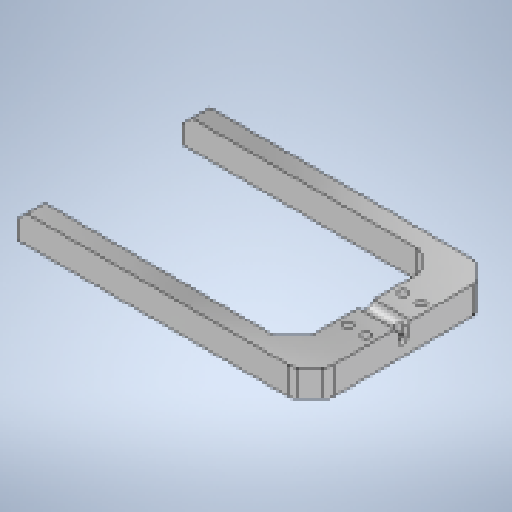
# Autodesk Inventor part: Rack
Saved by Autodesk Inventor 2023.2 (Build 272271000, 271)
## iProperties
Created: 2024-01-11
Part Number: Rack
Material: Aluminum 6061
Document SubType Name: Modeling
Designer: Nathan Cai
Mass: 47.5028 g
Surface Area: 86.9372 cm^2
Volume: 17.5936 cm^3
Density: 2.7 g/cm^3
Appearance: Aluminum - Flat
Author: Nathan Cai
Autodesk Inventor part; units mm, degrees
ref_plane "YZ Plane" through (0, 0, 0) normal (1, 0, 0) x (0, 1, 0)
ref_plane "XZ Plane" through (0, 0, 0) normal (0, 1, 0) x (-1, 0, 0)
ref_plane "XY Plane" through (0, 0, 0) normal (0, 0, 1) x (1, 0, 0)
sketch "Sketch1" plane through (0, 0, 0) normal (0, 1, 0) x (-1, 0, 0)
  line L0 (44.45, 23.8125) -> (-44.45, 23.8125)
  line L1 (-44.45, 23.8125) -> (-44.45, -23.8125)
  line L2 (-44.45, -23.8125) -> (44.45, -23.8125)
  line L3 (44.45, -23.8125) -> (44.45, 23.8125)
  line L4 (44.45, 23.8125) -> (-44.45, -23.8125) construction
  line L5 (-44.45, 23.8125) -> (44.45, -23.8125) construction
  line L6 (0, 0) -> (-44.45, 0) construction
  line L7 (44.45, 30.1625) -> (-57.15, 30.1625)
  line L8 (-57.15, 30.1625) -> (-57.15, -30.1625)
  line L9 (-57.15, -30.1625) -> (44.45, -30.1625)
  line L10 (44.45, -30.1625) -> (44.45, 30.1625)
  line L11 (44.45, 30.1625) -> (-57.15, -30.1625) construction
  line L12 (-57.15, 30.1625) -> (44.45, -30.1625) construction
  point P0 (-6.35, 0)
  point P1 (44.45, 23.8125)
  dimension "d0" = 88.9
  dimension "d1" = 47.625
  dimension "d2" = 6.35
  dimension "d3" = 12.7
  constraints: 26 end point, 5 midpoint, 4 parallel, 2 horizontal, 2 perpendicular, 2 point on line
  measures "d0" distance of L2.end L1.end
  measures "d1" distance of L1.end L0.end
  measures "d2" distance between parallel lines of L2 L9
  measures "d3" distance between parallel lines of L1 L8
extrude "Extrusion1" add sketch "Sketch1" along normal blind 9.525 contours L0 L1 L2 L10 L9 L8 L7
chamfer "Chamfer1" distance 6.35 angle 45 4 edges at (44.45, 4.7625, 23.8125) (57.15, 4.7625, 30.1625) (44.45, 4.7625, -23.8125) (57.15, 4.7625, -30.1625)
fillet "Fillet1" radius 3.175 8 edges at (38.1, 4.7625, 23.8125) (44.45, 4.7625, 17.4625) (44.45, 4.7625, -17.4625) (38.1, 4.7625, -23.8125) (50.8, 4.7625, -30.1625) (57.15, 4.7625, -23.8125) (57.15, 4.7625, 23.8125) (50.8, 4.7625, 30.1625)
sketch "Sketch2" plane through (57.15, 0, 22.4974) normal (1, 0, 0) x (0, 0, -1)
  line L0 (38.6447, 9.525) -> (6.35, 9.525) projected
  line L1 (22.4974, 9.525) -> (22.4974, 0) construction
  line L2 (38.6447, 0) -> (6.35, 0) projected
  circle A0 centre (22.4974, 4.7625) radius 3.175 construction
  circle A1 centre (22.4974, 11.1125) radius 3.175
  line L3 (22.4974, 17.1125) -> (22.4974, 5.1125) construction
  line L4 (20.9974, 17.1125) -> (20.9974, 5.1125)
  line L5 (23.9974, 5.1125) -> (23.9974, 17.1125)
  arc A2 (23.9974, 17.1125) -> (20.9974, 17.1125) centre (22.4974, 17.1125) ccw
  arc A3 (20.9974, 5.1125) -> (23.9974, 5.1125) centre (22.4974, 5.1125) ccw
  point P0 (19.7477, 9.525)
  point P1 (25.247, 9.525)
  point P2 (23.9974, 8.3142)
  point P3 (20.9974, 8.3142)
  dimension "d10" = 6.35
  dimension "d20" = 6.35
  dimension "d21" = 6.35
  dimension "d22" = 3
  dimension "d23" = 12
  constraints: 10 end point, 4 centre point, 4 point on circle, 4 tangent, 3 midpoint, 2 point on line, 1 parallel, 1 perpendicular
  measures "d10" diameter of A0
  measures "d20" diameter of A1
  measures "d21" distance of A0.centre A1.centre
  measures "d22" diameter of A3
  measures "d23" distance of L3.end L3.start
sketch "Sketch4" plane through (0, 9.525, 0) normal (0, 1, 0) x (1, 0, 0)
  line L0 (44.45, 16.1474) -> (44.45, -16.1474) projected
  line L1 (44.45, 0) -> (57.15, 0) construction
  line L2 (57.15, -22.4974) -> (57.15, 22.4974) projected
  line L3 (47.625, -9.525) -> (53.975, -9.525) construction
  line L4 (53.975, -9.525) -> (53.975, 9.525) construction
  line L5 (53.975, 9.525) -> (47.625, 9.525) construction
  line L6 (47.625, 9.525) -> (47.625, -9.525) construction
  line L7 (47.625, -9.525) -> (53.975, 9.525) construction
  line L8 (53.975, -9.525) -> (47.625, 9.525) construction
  circle A0 centre (47.625, -9.525) radius 1.5
  circle A1 centre (47.625, 9.525) radius 1.5
  circle A2 centre (53.975, -9.525) radius 1.5
  circle A3 centre (53.975, 9.525) radius 1.5
  point P0 (0, 0)
  point P1 (50.8, 0)
  dimension "d27" = 6.35
  dimension "d28" = 19.05
  dimension "d29" = 3
  dimension "d32" = 19.05
  dimension "d35" = 6.35
  constraints: 14 end point, 5 midpoint, 4 centre point, 2 horizontal, 2 parallel, 1 coincident, 1 perpendicular, 1 vertical, 6 other
  measures "d27" distance of L5.end L4.end
  measures "d28" distance of L4.end L3.end
  measures "d29" diameter of A0
  measures "d32" distance of A0.centre A1.centre
  measures "d35" distance of A0.centre A2.centre
extrude "Extrusion5" cut sketch "Sketch4" against normal through all
extrude "Extrusion2" cut sketch "Sketch2" against normal through all contours A1 L5 L0 | L5 A1 L4 L0 | L4 A1 L0 picked at (24.7175, 9.3654) picked at (22.4974, 8.9958) picked at (20.2773, 9.3654)
extrude "Extrusion4" cut sketch "Sketch2" against normal blind 3 contours L5 A3 L4 A1
fillet "Fillet3" radius 1.5 3 edges at (54.15, 6.7133, 1.5) (54.15, 6.7133, -1.5) (54.15, 3.6125, 0)
chamfer "Chamfer2" distance 3.175 angle 45 2 edges at (-44.45, 9.525, -26.9875) (-44.45, 9.525, 26.9875)
equation "\"d32\" = d28"
equation "\"d35\" = d27"
body "Solid1"
